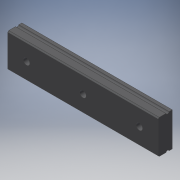
# Autodesk Inventor part: SEBS 9WA UU1T1-80P
Saved by Autodesk Inventor 2018.2 (Build 222227000, 227)
## iProperties
Category: PARTsolutions
Company: NB LINEAR
Created: 2015-08-08
Part Number: SEBS 9WA UU1T1-80P
Catalog Web Link: www.cadenas.de
Description: LINEAR BEARING, WIDE BLOCK, 80MM RAIL
Vendor: NB LINEAR
Document SubType Name: Modeling
Designer: PARTuser1
Manufacturer: NIPPON_BR
Mass: 10.1732 g
Surface Area: 46.8297 cm^2
Volume: 10.1732 cm^3
Density: 1 g/cm^3
Material: Generic
Appearance: PSOLRGB-192-192-192
PSOL_IDENT_0: {$CADENAS_DATA\23d-libs\nippon_br\slide_guide\seb_a\sebs-wa_way\sebs-wa_way_rail.prj},232 {VTYP=3D},
PSOL_IDENT_1: {NB=SEBSSEBS 9WA9WA18010 Track},{LINA=SEBS 9WA1-80},{NN=wide blocks, SEBS-WA/WAY R},{DATE=24.03.2015
PSOL_IDENT_2: 13:55:45},{GEOMDATE=24.03.2015 13:55:00},{VERSION=},{LINEID=170},{LINESUBID=-1},{WBVAR=SPC,S,NOB,TO
PSOL_IDENT_3: P,SS,LOR,TOR,TON,N1}  {NB=SEBSSEBS 9WA9WA18010 Track},{LINA=SEBS 9WA1-80},{KT=DUMMY},{SPC=SEBS},{S=9
PSOL_IDENT_4: WA},{NOB=1},{TOP=},{SS=},{LOR=80},{TOR=},{TON=},{N1=10},{N22=10},{NXMIN=0.25},{NXMAX=26},{PN=SEBS 9W
PSOL_IDENT_5: A},{W=6.000},{B=30.000},{BB=9.000},{H1=7.500},{TOP1='','Standard'},{UD=18.000},{UD1=7.500},{CF1=0.57
PSOL_IDENT_6: 0},{UD2=4.140},{UD3=5.860},{UD4=0.650},{S12='9WA','9WA'},{LMIN=50},{LMAX=1480},{D=3.500},{G=6.000},{
PSOL_IDENT_7: H=4.500},{N=10.000},{ND2='9WAS'},{P=30.000},{NDM=4.000},{KDM=3.242},{SS1='', 'No seal', 'UU', 'with
PSOL_IDENT_8: Side Seal (UU)'},{NMIN=4.000},{NMAX=26},{EK=20},{M=2},{A=20},{N1X=10},{N2X=26},{N1MAX=16},{N1MIN=-6}
PSOL_IDENT_9: ,{AX=10},{CF=0.000},{UDT=3.000},{SPC1='SEBS','Antocorrosion (SEBS)'},{R=0.900},{R1=9.250},{R2=5.000}
PSOL_IDENT_10: ,{C=18.000}
NN: wide blocks, SEBS-WA/WAY R
NB: SEBSSEBS 9WA9WA18010 Track
NBSYN: $SPC.$PN.$TOP.$S.$NOB.$SS.$LOR.$TOR.$TON.$N1. Track
LINA: SEBS 9WA1-80
SPC: Antocorrosion (SEBS)
S: 9WA
NOB: 1
TOP: Standard
SS: No seal
LOR: 80.0
TOR: Counterbore
TON: Symmetry
N1: 10.00
PN: SEBS 9WA
W: 6.000
B: 30.000
BB: 9.000
H1: 7.500
UD: 18.000
UD1: 7.500
CF1: 0.570
UD2: 4.140
UD3: 5.860
UD4: 0.650
D: 3.500
G: 6.000
H: 4.500
N: 10.000
ND2: '9WAS'
P: 30.000
NDM: 4.000
KDM: 3.242
NMIN: 4.000
CF: 0.000
UDT: 3.000
R: 0.900
R1: 9.250
R2: 5.000
C: 18.000
SUPPLIER: NIPPON_BR
ARTICLENO: SEBSSEBS 9WA9WA18010 Track
BOMINFO: SEBS 9WA1-80
CREATOR: CADENAS GmbH
ALTERED ITEM DESCRIPTION: N/A
ALTERED ITEM PART NUMBER: N/A
ALTERED ITEM VENDOR: N/A
DESIGN DEPARTMENT: HHMI: JRC - ID&F
Title: SEBS 9WA1-80
Author: Cadenas PARTsolutions
Revision Number: 0
Autodesk Inventor part; units mm, degrees
sketch "Sketch_1" plane through (-10, 0, 0) normal (1, 0, 0) x (0, 0, -1)
  arc A0 (-9, 4.1354) -> (-9, 5.8646) centre (-9.25, 5) ccw
  line L0 (-9, 4.1354) -> (-9, 0.57)
  line L1 (-9, 0.57) -> (-8.43, 0)
  line L2 (-8.43, 0) -> (8.43, 0)
  line L3 (8.43, 0) -> (9, 0.57)
  line L4 (9, 0.57) -> (9, 4.1354)
  arc A1 (9, 5.8646) -> (9, 4.1354) centre (9.25, 5) ccw
  line L5 (9, 5.8646) -> (9, 7.5)
  line L6 (9, 7.5) -> (-9, 7.5)
  line L7 (-9, 7.5) -> (-9, 5.8646)
  constraints: 16 end point, 4 point on circle, 2 centre point
extrude "Extrusion1" add sketch "Sketch_1" along normal blind 80
sketch "Sketch2" plane through (-10, 7.5, 9) normal (0, 1, 0) x (1, 0, 0)
  point P0 (10, 9)
hole "Hole1" at (0, 7.5, 0) direction (0, -1, 0) diameter 3.5 depth 7.5 counterbore diameter 6 counterbore depth 4.5
pattern_linear "Rectangular Pattern1" count 3 spacing 30 along (1, 0, 0) of "Hole1"
ref_plane "rail_XY" through (-10, 0, 0) normal (1, 0, 0) x (0, 0, -1)
ref_plane "rail_YZ" through (-10, 0, 0) normal (0, 0, -1) x (0, 1, 0)
ref_plane "rail_ZX" through (-10, 0, 0) normal (0, 1, 0) x (1, 0, 0)
body "Solid1"
